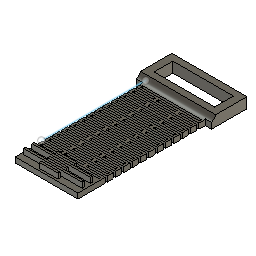
base_comp12 (Autodesk Fusion 360 design; units mm, degrees)
Autodesk Fusion 360 part; units mm, degrees
note: some values were not read from the file. Set by a fixed rule: which face or edge a step refers to.
(part 1 of 3)
sketch "Sketch1" plane through (0, 0, 0) normal (0, 0, 1) x (1, 0, 0)
  line L0 (-25, 25) -> (35, 25)
  line L1 (35, 25) -> (35, -145)
  line L2 (35, -145) -> (-25, -145)
  line L3 (-25, -145) -> (-25, 25)
  dimension "d1" = 60
  dimension "d2" = 170
  constraint perpendicular L0 L1
  constraint parallel L0 L2
  constraint parallel L1 L3
  constraint horizontal L0
  measures "d1" distance of L0.start L0.end
  measures "d2" distance of L0.start L2.end
extrude "Extrude1" add sketch "Sketch1" along normal blind 5
sketch "Sketch2" plane through (0, 0, 5) normal (0, 0, 1) x (-1, 0, 0)
  line L0 (25, 145) -> (-35, 145)
  line L1 (-35, 145) -> (-35, -25)
  line L2 (-35, -25) -> (25, -25)
  line L3 (25, -25) -> (25, 145)
  line L4 (25, -24) -> (25, -22)
  line L5 (25, -22) -> (7, -22)
  line L6 (7, -22) -> (7, -24)
  line L7 (7, -24) -> (25, -24)
  line L8 (4, -24) -> (4, -22)
  line L9 (4, -22) -> (-14, -22)
  line L10 (-14, -22) -> (-14, -24)
  line L11 (-14, -24) -> (4, -24)
  line L12 (-17, -24) -> (-17, -22)
  line L13 (-17, -22) -> (-35, -22)
  line L14 (-35, -22) -> (-35, -24)
  line L15 (-35, -24) -> (-17, -24)
  line L16 (-17, -22) -> (-35, -22)
  line L17 (-17, -24) -> (-17, -22)
  line L18 (25, -22) -> (7, -22)
  line L19 (7, -22) -> (7, -24)
  line L20 (-35, -24) -> (-17, -24)
  line L21 (4, -24) -> (4, -22)
  line L22 (-35, -22) -> (-35, -24)
  line L23 (25, -24) -> (25, -22)
  line L24 (4, -22) -> (-14, -22)
  line L25 (-14, -24) -> (4, -24)
  line L26 (-14, -22) -> (-14, -24)
  line L27 (7, -24) -> (25, -24)
  dimension "d5" = 2
  dimension "d6" = 18
  dimension "d7" = 2
  dimension "d8" = 18
  dimension "d9" = 2
  dimension "d10" = 18
  dimension "d11" = 2
  dimension "d12" = 18
  dimension "d13" = 2
  dimension "d14" = 18
  dimension "d15" = 2
  dimension "d16" = 18
  constraint perpendicular L4 L5
  constraint parallel L4 L6
  constraint parallel L5 L7
  constraint perpendicular L2 L4
  constraint coincident L3 L4.start
  constraint perpendicular L8 L9
  constraint parallel L8 L10
  constraint parallel L9 L11
  constraint perpendicular L5 L8
  constraint perpendicular L12 L13
  constraint parallel L12 L14
  constraint parallel L13 L15
  constraint parallel L1 L12
  constraint perpendicular L18 L23
  constraint parallel L19 L23
  constraint parallel L18 L27
  constraint perpendicular L21 L24
  constraint parallel L21 L26
  constraint parallel L24 L25
  constraint perpendicular L18 L21
  constraint perpendicular L16 L17
  constraint parallel L17 L22
  constraint parallel L16 L20
  measures "d5" distance of L4.start L4.end
  measures "d6" distance of L4.start L6.end
  measures "d7" distance of L8.start L8.end
  measures "d8" distance of L8.start L10.end
  measures "d9" distance of L12.start L12.end
  measures "d10" distance of L12.start L14.end
  measures "d11" distance of L4.start L4.end
  measures "d12" distance of L4.start L6.end
  measures "d13" distance of L8.end L8.start
  measures "d14" distance of L10.end L8.start
  measures "d15" distance of L12.end L12.start
  measures "d16" distance of L14.end L12.start
sketch "Sketch3" plane through (0, 0, 5) normal (0, 0, 1) x (-1, 0, 0)
  line L0 (23, -20) -> (23, -18)
  line L1 (23, -18) -> (-33, -18)
  line L2 (-33, -18) -> (-33, -20)
  line L3 (-33, -20) -> (23, -20)
  dimension "d17" = 2
  dimension "d18" = 56
  constraint perpendicular L0 L1
  constraint parallel L0 L2
  constraint parallel L1 L3
  constraint vertical L0
  measures "d17" distance of L0.start L0.end
  measures "d18" distance of L0.start L2.end
sketch "Sketch4" plane through (0, 0, 5) normal (0, 0, 1) x (-1, 0, 0)
extrude "Extrude2" cut sketch "Sketch3" against normal blind 11
extrude "Extrude3" cut sketch "Sketch2" against normal blind 26 contours L3 L4 L5 L6 L7 L18 L19 L23 L27 | L1 L12 L13 L14 L15 L16 L17 L20 L22 | L8 L9 L10 L11 L21 L24 L25 L26
sketch "Sketch5" plane through (0, 0, 5) normal (0, 0, 1) x (-1, 0, 0)
  line L0 (-17, -24) -> (-35, -24)
  line L1 (-35, -24) -> (-35, -25)
  line L2 (-35, -25) -> (25, -25)
  line L3 (25, -25) -> (25, -24)
  line L4 (25, -24) -> (7, -24)
  line L5 (7, -24) -> (7, -22)
  line L6 (7, -22) -> (25, -22)
  line L7 (25, -22) -> (25, 145)
  line L8 (25, 145) -> (-35, 145)
  line L9 (-35, 145) -> (-35, -22)
  line L10 (-35, -22) -> (-17, -22)
  line L11 (-17, -22) -> (-17, -24)
  line L12 (4, -24) -> (-14, -24)
  line L13 (-14, -24) -> (-14, -22)
  line L14 (-14, -22) -> (4, -22)
  line L15 (4, -22) -> (4, -24)
  line L16 (23, -18) -> (23, -20)
  line L17 (23, -20) -> (-33, -20)
  line L18 (-33, -20) -> (-33, -18)
  line L19 (-33, -18) -> (23, -18)
  line L20 (25, -16) -> (25, -14)
  line L21 (25, -14) -> (7, -14)
  line L22 (7, -14) -> (7, -16)
  line L23 (7, -16) -> (25, -16)
  line L24 (4, -16) -> (4, -14)
  line L25 (4, -14) -> (-14, -14)
  line L26 (-14, -14) -> (-14, -16)
  line L27 (-14, -16) -> (4, -16)
  line L28 (-17, -16) -> (-17, -14)
  line L29 (-17, -14) -> (-35, -14)
  line L30 (-35, -14) -> (-35, -16)
  line L31 (-35, -16) -> (-17, -16)
  line L32 (23, -12) -> (23, -10)
  line L33 (23, -10) -> (-33, -10)
  line L34 (-33, -10) -> (-33, -12)
  line L35 (-33, -12) -> (23, -12)
  line L36 (25, -8) -> (25, -6)
  line L37 (25, -6) -> (7, -6)
  line L38 (7, -6) -> (7, -8)
  line L39 (7, -8) -> (25, -8)
  line L40 (4, -8) -> (4, -6)
  line L41 (4, -6) -> (-14, -6)
  line L42 (-14, -6) -> (-14, -8)
  line L43 (-14, -8) -> (4, -8)
  line L44 (-17, -8) -> (-17, -6)
  line L45 (-17, -6) -> (-35, -6)
  line L46 (-35, -6) -> (-35, -8)
  line L47 (-35, -8) -> (-17, -8)
  line L48 (23, -4) -> (23, -2)
  line L49 (23, -2) -> (-33, -2)
  line L50 (-33, -2) -> (-33, -4)
  line L51 (-33, -4) -> (23, -4)
  line L52 (25, 0) -> (25, 2)
  line L53 (25, 2) -> (7, 2)
  line L54 (7, 2) -> (7, 0)
  line L55 (7, 0) -> (25, 0)
  line L56 (4, 0) -> (4, 2)
  line L57 (4, 2) -> (-14, 2)
  line L58 (-14, 2) -> (-14, 0)
  line L59 (-14, 0) -> (4, 0)
  line L60 (-17, 0) -> (-17, 2)
  line L61 (-17, 2) -> (-35, 2)
  line L62 (-35, 2) -> (-35, 0)
  line L63 (-35, 0) -> (-17, 0)
  line L64 (23, 4) -> (23, 6)
  line L65 (23, 6) -> (-33, 6)
  line L66 (-33, 6) -> (-33, 4)
  line L67 (-33, 4) -> (23, 4)
  line L68 (25, 8) -> (25, 10)
  line L69 (25, 10) -> (7, 10)
  line L70 (7, 10) -> (7, 8)
  line L71 (7, 8) -> (25, 8)
  line L72 (4, 8) -> (4, 10)
  line L73 (4, 10) -> (-14, 10)
  line L74 (-14, 10) -> (-14, 8)
  line L75 (-14, 8) -> (4, 8)
  line L76 (-17, 8) -> (-17, 10)
  line L77 (-17, 10) -> (-35, 10)
  line L78 (-35, 10) -> (-35, 8)
  line L79 (-35, 8) -> (-17, 8)
  line L80 (23, 12) -> (23, 14)
  line L81 (23, 14) -> (-33, 14)
  line L82 (-33, 14) -> (-33, 12)
  line L83 (-33, 12) -> (23, 12)
  line L84 (25, 16) -> (25, 18)
  line L85 (25, 18) -> (7, 18)
  line L86 (7, 18) -> (7, 16)
  line L87 (7, 16) -> (25, 16)
  line L88 (4, 16) -> (4, 18)
  line L89 (4, 18) -> (-14, 18)
  line L90 (-14, 18) -> (-14, 16)
  line L91 (-14, 16) -> (4, 16)
  line L92 (-17, 16) -> (-17, 18)
  line L93 (-17, 18) -> (-35, 18)
  line L94 (-35, 18) -> (-35, 16)
  line L95 (-35, 16) -> (-17, 16)
  line L96 (23, 20) -> (23, 22)
  line L97 (23, 22) -> (-33, 22)
  line L98 (-33, 22) -> (-33, 20)
  line L99 (-33, 20) -> (23, 20)
  line L100 (25, 24) -> (25, 26)
  line L101 (25, 26) -> (7, 26)
  line L102 (7, 26) -> (7, 24)
  line L103 (7, 24) -> (25, 24)
  line L104 (4, 24) -> (4, 26)
  line L105 (4, 26) -> (-14, 26)
  line L106 (-14, 26) -> (-14, 24)
  line L107 (-14, 24) -> (4, 24)
  line L108 (-17, 24) -> (-17, 26)
  line L109 (-17, 26) -> (-35, 26)
  line L110 (-35, 26) -> (-35, 24)
  line L111 (-35, 24) -> (-17, 24)
  line L112 (23, 28) -> (23, 30)
  line L113 (23, 30) -> (-33, 30)
  line L114 (-33, 30) -> (-33, 28)
  line L115 (-33, 28) -> (23, 28)
  line L116 (25, 32) -> (7, 32)
  line L117 (7, 32) -> (7, 34)
  line L118 (7, 34) -> (25, 34)
  line L119 (25, 34) -> (25, 32)
  line L120 (4, 32) -> (4, 34)
  line L121 (4, 34) -> (-14, 34)
  line L122 (-14, 34) -> (-14, 32)
  line L123 (-14, 32) -> (4, 32)
  line L124 (-17, 32) -> (-17, 34)
  line L125 (-17, 34) -> (-35, 34)
  line L126 (-35, 34) -> (-35, 32)
  line L127 (-35, 32) -> (-17, 32)
  line L128 (23, 36) -> (23, 38)
  line L129 (23, 38) -> (-33, 38)
  line L130 (-33, 38) -> (-33, 36)
  line L131 (-33, 36) -> (23, 36)
  dimension "d23" = 2
  dimension "d24" = 18
  dimension "d25" = 18
  dimension "d26" = 18
  dimension "d27" = 2
  dimension "d28" = 56
  dimension "d29" = 2
  dimension "d30" = 18
  dimension "d31" = 18
  dimension "d32" = 18
  dimension "d33" = 56
  dimension "d34" = 2
  dimension "d35" = 18
  dimension "d36" = 2
  dimension "d37" = 18
  dimension "d38" = 2
  dimension "d39" = 56
  dimension "d40" = 18
  dimension "d41" = 18
  dimension "d42" = 2
  dimension "d43" = 18
  dimension "d44" = 56
  dimension "d45" = 2
  dimension "d46" = 18
  dimension "d47" = 2
  dimension "d48" = 18
  dimension "d49" = 2
  dimension "d50" = 18
  dimension "d51" = 2
  dimension "d52" = 56
  dimension "d53" = 2
  dimension "d54" = 18
  dimension "d55" = 2
  dimension "d56" = 18
  dimension "d57" = 2
  dimension "d58" = 18
  dimension "d59" = 2
  dimension "d60" = 56
  dimension "d61" = 2
  dimension "d62" = 18
  dimension "d63" = 2
  dimension "d64" = 18
  dimension "d65" = 56
  constraint perpendicular L20 L21
  constraint parallel L20 L22
  constraint parallel L21 L23
  constraint parallel L7 L20
  constraint coincident L7 L20.start
  constraint perpendicular L24 L25
  constraint parallel L24 L26
  constraint parallel L25 L27
  constraint vertical L24
  constraint perpendicular L28 L29
  constraint parallel L28 L30
  constraint parallel L29 L31
  constraint perpendicular L27 L28
  constraint perpendicular L32 L33
  constraint parallel L32 L34
  constraint parallel L33 L35
  constraint vertical L32
  constraint perpendicular L36 L37
  constraint parallel L36 L38
  constraint parallel L37 L39
  constraint perpendicular L33 L36
  constraint coincident L7 L36.start
  constraint perpendicular L40 L41
  constraint parallel L40 L42
  constraint parallel L41 L43
  constraint perpendicular L33 L40
  constraint perpendicular L44 L45
  constraint parallel L44 L46
  constraint parallel L45 L47
  constraint perpendicular L41 L44
  constraint perpendicular L48 L49
  constraint parallel L48 L50
  constraint parallel L49 L51
  constraint perpendicular L37 L48
  constraint perpendicular L52 L53
  constraint parallel L52 L54
  constraint parallel L53 L55
  constraint perpendicular L45 L52
  constraint coincident L7 L52.start
  constraint perpendicular L56 L57
  constraint parallel L56 L58
  constraint parallel L57 L59
  constraint vertical L56
  constraint perpendicular L60 L61
  constraint parallel L60 L62
  constraint parallel L61 L63
  constraint vertical L60
  constraint perpendicular L64 L65
  constraint parallel L64 L66
  constraint parallel L65 L67
  constraint vertical L64
  constraint perpendicular L68 L69
  constraint parallel L68 L70
  constraint parallel L69 L71
  constraint coincident L7 L68.end
  constraint coincident L7 L68.start
  constraint perpendicular L72 L73
  constraint parallel L72 L74
  constraint parallel L73 L75
  constraint perpendicular L71 L72
  constraint perpendicular L76 L77
  constraint parallel L76 L78
  constraint parallel L77 L79
  constraint perpendicular L73 L76
  constraint perpendicular L80 L81
  constraint parallel L80 L82
  constraint parallel L81 L83
  constraint perpendicular L71 L80
  constraint perpendicular L84 L85
  constraint parallel L84 L86
  constraint parallel L85 L87
  constraint perpendicular L73 L84
  constraint coincident L7 L84.start
  constraint perpendicular L88 L89
  constraint parallel L88 L90
  constraint parallel L89 L91
  constraint perpendicular L85 L88
  constraint perpendicular L92 L93
  constraint parallel L92 L94
  constraint parallel L93 L95
  constraint perpendicular L81 L92
  constraint perpendicular L96 L97
  constraint parallel L96 L98
  constraint parallel L97 L99
  constraint perpendicular L85 L96
  constraint perpendicular L100 L101
  constraint parallel L100 L102
  constraint parallel L101 L103
  constraint perpendicular L97 L100
  constraint coincident L7 L100.start
  constraint perpendicular L104 L105
  constraint parallel L104 L106
  constraint parallel L105 L107
  constraint perpendicular L101 L104
  constraint perpendicular L108 L109
  constraint parallel L108 L110
  constraint parallel L109 L111
  constraint perpendicular L105 L108
  constraint perpendicular L112 L113
  constraint parallel L112 L114
  constraint parallel L113 L115
  constraint perpendicular L101 L112
  constraint horizontal L116
  constraint vertical L117
  constraint horizontal L118
  constraint vertical L119
  constraint coincident L7 L116.start
  constraint perpendicular L120 L121
  constraint parallel L120 L122
  constraint parallel L121 L123
  constraint perpendicular L113 L120
  constraint perpendicular L124 L125
  constraint parallel L124 L126
  constraint parallel L125 L127
  constraint perpendicular L121 L124
  constraint perpendicular L128 L129
  constraint parallel L128 L130
  constraint parallel L129 L131
  constraint perpendicular L118 L128
  measures "d23" distance of L20.start L20.end
  measures "d24" distance of L20.start L22.end
  measures "d25" distance of L24.start L26.end
  measures "d26" distance of L28.start L30.end
  measures "d27" distance of L32.start L32.end
  measures "d28" distance of L32.start L34.end
  measures "d29" distance of L36.start L36.end
  measures "d30" distance of L36.start L38.end
  measures "d31" distance of L40.start L42.end
  measures "d32" distance of L44.start L46.end
  measures "d33" distance of L48.start L50.end
  measures "d34" distance of L52.start L52.end
  measures "d35" distance of L52.start L54.end
  measures "d36" distance of L56.start L56.end
  measures "d37" distance of L56.start L58.end
  measures "d38" distance of L64.start L64.end
  measures "d39" distance of L64.start L66.end
  measures "d40" distance of L68.start L70.end
  measures "d41" distance of L72.start L74.end
  measures "d42" distance of L76.start L76.end
  measures "d43" distance of L76.start L78.end
  measures "d44" distance of L80.start L82.end
  measures "d45" distance of L84.start L84.end
  measures "d46" distance of L84.start L86.end
  measures "d47" distance of L88.start L88.end
  measures "d48" distance of L88.start L90.end
  measures "d49" distance of L92.start L92.end
  measures "d50" distance of L92.start L94.end
  measures "d51" distance of L96.start L96.end
  measures "d52" distance of L96.start L98.end
  measures "d53" distance of L100.start L100.end
  measures "d54" distance of L100.start L102.end
  measures "d55" distance of L104.start L104.end
  measures "d56" distance of L104.start L106.end
  measures "d57" distance of L108.start L108.end
  measures "d58" distance of L108.start L110.end
  measures "d59" distance of L112.start L112.end
  measures "d60" distance of L112.start L114.end
  measures "d61" distance of L120.start L120.end
  measures "d62" distance of L120.start L122.end
  measures "d63" distance of L124.start L124.end
  measures "d64" distance of L124.start L126.end
  measures "d65" distance of L128.start L130.end
extrude "Extrude4" cut sketch "Sketch5" against normal blind 35 contours L9 L28 L29 L30 L31 | L9 L44 L45 L46 L47 | L9 L60 L61 L62 L63 | L7 L20 L21 L22 L23 | L9 L76 L77 L78 L79 | L7 L36 L37 L38 L39 | L9 L92 L93 L94 L95 | L7 L52 L53 L54 L55 | L9 L108 L109 L110 L111 | L7 L68 L69 L70 L71 | L9 L124 L125 L126 L127 | L7 L84 L85 L86 L87 | L7 L100 L101 L102 L103 | L7 L116 L117 L118 L119 | L12 L13 L14 L15 | L16 L17 L18 L19 | L24 L25 L26 L27 | L32 L33 L34 L35 | L40 L41 L42 L43 | L48 L49 L50 L51 | L56 L57 L58 L59 | L64 L65 L66 L67 | L72 L73 L74 L75 | L80 L81 L82 L83 | L88 L89 L90 L91 | L96 L97 L98 L99 | L104 L105 L106 L107 | L112 L113 L114 L115 | L120 L121 L122 L123 | L128 L129 L130 L131
sketch "Sketch6" plane through (0, 0, 5) normal (0, 0, 1) x (-1, 0, 0)
  line L0 (25, 16) -> (7, 16)
  line L1 (7, 16) -> (7, 18)
  line L2 (7, 18) -> (25, 18)
  line L3 (25, 18) -> (25, 24)
  line L4 (25, 24) -> (7, 24)
  line L5 (7, 24) -> (7, 26)
  line L6 (7, 26) -> (25, 26)
  line L7 (25, 26) -> (25, 32)
  line L8 (25, 32) -> (7, 32)
  line L9 (7, 32) -> (7, 34)
  line L10 (7, 34) -> (25, 34)
  line L11 (25, 34) -> (25, 145)
  line L12 (25, 145) -> (-35, 145)
  line L13 (-35, 145) -> (-35, 34)
  line L14 (-35, 34) -> (-17, 34)
  line L15 (-17, 34) -> (-17, 32)
  line L16 (-17, 32) -> (-35, 32)
  line L17 (-35, 32) -> (-35, 26)
  line L18 (-35, 26) -> (-17, 26)
  line L19 (-17, 26) -> (-17, 24)
  line L20 (-17, 24) -> (-35, 24)
  line L21 (-35, 24) -> (-35, 18)
  line L22 (-35, 18) -> (-17, 18)
  line L23 (-17, 18) -> (-17, 16)
  line L24 (-17, 16) -> (-35, 16)
  line L25 (-35, 16) -> (-35, 10)
  line L26 (-35, 10) -> (-17, 10)
  line L27 (-17, 10) -> (-17, 8)
  line L28 (-17, 8) -> (-35, 8)
  line L29 (-35, 8) -> (-35, 2)
  line L30 (-35, 2) -> (-17, 2)
  line L31 (-17, 2) -> (-17, 0)
  line L32 (-17, 0) -> (-35, 0)
  line L33 (-35, 0) -> (-35, -6)
  line L34 (-35, -6) -> (-17, -6)
  line L35 (-17, -6) -> (-17, -8)
  line L36 (-17, -8) -> (-35, -8)
  line L37 (-35, -8) -> (-35, -14)
  line L38 (-35, -14) -> (-17, -14)
  line L39 (-17, -14) -> (-17, -16)
  line L40 (-17, -16) -> (-35, -16)
  line L41 (-35, -16) -> (-35, -22)
  line L42 (-35, -22) -> (-17, -22)
  line L43 (-17, -22) -> (-17, -24)
  line L44 (-17, -24) -> (-35, -24)
  line L45 (-35, -24) -> (-35, -25)
  line L46 (-35, -25) -> (25, -25)
  line L47 (25, -25) -> (25, -24)
  line L48 (25, -24) -> (7, -24)
  line L49 (7, -24) -> (7, -22)
  line L50 (7, -22) -> (25, -22)
  line L51 (25, -22) -> (25, -16)
  line L52 (25, -16) -> (7, -16)
  line L53 (7, -16) -> (7, -14)
  line L54 (7, -14) -> (25, -14)
  line L55 (25, -14) -> (25, -8)
  line L56 (25, -8) -> (7, -8)
  line L57 (7, -8) -> (7, -6)
  line L58 (7, -6) -> (25, -6)
  line L59 (25, -6) -> (25, 0)
  line L60 (25, 0) -> (7, 0)
  line L61 (7, 0) -> (7, 2)
  line L62 (7, 2) -> (25, 2)
  line L63 (25, 2) -> (25, 8)
  line L64 (25, 8) -> (7, 8)
  line L65 (7, 8) -> (7, 10)
  line L66 (7, 10) -> (25, 10)
  line L67 (25, 10) -> (25, 16)
  line L68 (23, -18) -> (23, -20)
  line L69 (23, -20) -> (-33, -20)
  line L70 (-33, -20) -> (-33, -18)
  line L71 (-33, -18) -> (23, -18)
  line L72 (4, -24) -> (-14, -24)
  line L73 (-14, -24) -> (-14, -22)
  line L74 (-14, -22) -> (4, -22)
  line L75 (4, -22) -> (4, -24)
  line L76 (23, 22) -> (23, 20)
  line L77 (23, 20) -> (-33, 20)
  line L78 (-33, 20) -> (-33, 22)
  line L79 (-33, 22) -> (23, 22)
  line L80 (23, 6) -> (23, 4)
  line L81 (23, 4) -> (-33, 4)
  line L82 (-33, 4) -> (-33, 6)
  line L83 (-33, 6) -> (23, 6)
  line L84 (23, -10) -> (23, -12)
  line L85 (23, -12) -> (-33, -12)
  line L86 (-33, -12) -> (-33, -10)
  line L87 (-33, -10) -> (23, -10)
  line L88 (4, -14) -> (4, -16)
  line L89 (4, -16) -> (-14, -16)
  line L90 (-14, -16) -> (-14, -14)
  line L91 (-14, -14) -> (4, -14)
  line L92 (4, -6) -> (4, -8)
  line L93 (4, -8) -> (-14, -8)
  line L94 (-14, -8) -> (-14, -6)
  line L95 (-14, -6) -> (4, -6)
  line L96 (4, 10) -> (4, 8)
  line L97 (4, 8) -> (-14, 8)
  line L98 (-14, 8) -> (-14, 10)
  line L99 (-14, 10) -> (4, 10)
  line L100 (4, 26) -> (4, 24)
  line L101 (4, 24) -> (-14, 24)
  line L102 (-14, 24) -> (-14, 26)
  line L103 (-14, 26) -> (4, 26)
  line L104 (4, 34) -> (4, 32)
  line L105 (4, 32) -> (-14, 32)
  line L106 (-14, 32) -> (-14, 34)
  line L107 (-14, 34) -> (4, 34)
  line L108 (4, 18) -> (4, 16)
  line L109 (4, 16) -> (-14, 16)
  line L110 (-14, 16) -> (-14, 18)
  line L111 (-14, 18) -> (4, 18)
  line L112 (4, 2) -> (4, 0)
  line L113 (4, 0) -> (-14, 0)
  line L114 (-14, 0) -> (-14, 2)
  line L115 (-14, 2) -> (4, 2)
  line L116 (23, 38) -> (23, 36)
  line L117 (23, 36) -> (-33, 36)
  line L118 (-33, 36) -> (-33, 38)
  line L119 (-33, 38) -> (23, 38)
  line L120 (23, -2) -> (23, -4)
  line L121 (23, -4) -> (-33, -4)
  line L122 (-33, -4) -> (-33, -2)
  line L123 (-33, -2) -> (23, -2)
  line L124 (23, 14) -> (23, 12)
  line L125 (23, 12) -> (-33, 12)
  line L126 (-33, 12) -> (-33, 14)
  line L127 (-33, 14) -> (23, 14)
  line L128 (23, 30) -> (23, 28)
  line L129 (23, 28) -> (-33, 28)
  line L130 (-33, 28) -> (-33, 30)
  line L131 (-33, 30) -> (23, 30)
  line L132 (25, 40) -> (25, 42)
  line L133 (25, 42) -> (7, 42)
  line L134 (7, 42) -> (7, 40)
  line L135 (7, 40) -> (25, 40)
  line L136 (4, 40) -> (4, 42)
  line L137 (4, 42) -> (-14, 42)
  line L138 (-14, 42) -> (-14, 40)
  line L139 (-14, 40) -> (4, 40)
  line L140 (-17, 40) -> (-17, 42)
  line L141 (-17, 42) -> (-35, 42)
  line L142 (-35, 42) -> (-35, 40)
  line L143 (-35, 40) -> (-17, 40)
  line L144 (23, 44) -> (23, 46.2715)
  line L145 (23, 46.2715) -> (-33, 46.2715)
  line L146 (-33, 46.2715) -> (-33, 44)
  line L147 (-33, 44) -> (23, 44)
  line L148 (25, 48) -> (7, 48)
  line L149 (7, 48) -> (7, 50)
  line L150 (7, 50) -> (25, 50)
  line L151 (25, 50) -> (25, 48)
  line L152 (4, 48) -> (4, 50)
  line L153 (4, 50) -> (-14, 50)
  line L154 (-14, 50) -> (-14, 48)
  line L155 (-14, 48) -> (4, 48)
  line L156 (-17, 48) -> (-17, 50)
  line L157 (-17, 50) -> (-35, 50)
  line L158 (-35, 50) -> (-35, 48)
  line L159 (-35, 48) -> (-17, 48)
  line L160 (23, 52) -> (23, 54)
  line L161 (23, 54) -> (-33, 54)
  line L162 (-33, 54) -> (-33, 52)
  line L163 (-33, 52) -> (23, 52)
  line L164 (25, 56) -> (25, 58)
  line L165 (25, 58) -> (7, 58)
  line L166 (7, 58) -> (7, 56)
  line L167 (7, 56) -> (25, 56)
  line L168 (4, 56) -> (4, 58)
  line L169 (4, 58) -> (-14, 58)
  line L170 (-14, 58) -> (-14, 56)
  line L171 (-14, 56) -> (4, 56)
  line L172 (-17, 56) -> (-17, 58)
  line L173 (-17, 58) -> (-35, 58)
  line L174 (-35, 58) -> (-35, 56)
  line L175 (-35, 56) -> (-17, 56)
  line L176 (23, 60) -> (23, 62)
  line L177 (23, 62) -> (-33, 62)
  line L178 (-33, 62) -> (-33, 60)
  line L179 (-33, 60) -> (23, 60)
  line L180 (25, 64) -> (25, 66)
  line L181 (25, 66) -> (7, 66)
  line L182 (7, 66) -> (7, 64)
  line L183 (7, 64) -> (25, 64)
  line L184 (4, 64) -> (4, 66)
  line L185 (4, 66) -> (-14, 66)
  line L186 (-14, 66) -> (-14, 64)
  line L187 (-14, 64) -> (4, 64)
  line L188 (-17, 64) -> (-17, 66)
  line L189 (-17, 66) -> (-35, 66)
  line L190 (-35, 66) -> (-35, 64)
  line L191 (-35, 64) -> (-17, 64)
  line L192 (23, 68) -> (23, 70)
  line L193 (23, 70) -> (-33, 70)
  line L194 (-33, 70) -> (-33, 68)
  line L195 (-33, 68) -> (23, 68)
  line L196 (25, 72) -> (25, 74)
  line L197 (25, 74) -> (7, 74)
  line L198 (7, 74) -> (7, 72)
  line L199 (7, 72) -> (25, 72)
  line L200 (4, 72) -> (4, 74)
  line L201 (4, 74) -> (-14, 74)
  line L202 (-14, 74) -> (-14, 72)
  line L203 (-14, 72) -> (4, 72)
  line L204 (-17, 72) -> (-17, 74)
  line L205 (-17, 74) -> (-35, 74)
  line L206 (-35, 74) -> (-35, 72)
  line L207 (-35, 72) -> (-17, 72)
  line L208 (23, 76) -> (23, 78)
  line L209 (23, 78) -> (-33, 78)
  line L210 (-33, 78) -> (-33, 76)
  line L211 (-33, 76) -> (23, 76)
  line L212 (25, 80) -> (25, 82)
  line L213 (25, 82) -> (7, 82)
  line L214 (7, 82) -> (7, 80)
  line L215 (7, 80) -> (25, 80)
  line L216 (4, 80) -> (4, 82)
  line L217 (4, 82) -> (-14, 82)
  line L218 (-14, 82) -> (-14, 80)
  line L219 (-14, 80) -> (4, 80)
  line L220 (-17, 80) -> (-17, 82)
  line L221 (-17, 82) -> (-35, 82)
  line L222 (-35, 82) -> (-35, 80)
  line L223 (-35, 80) -> (-17, 80)
  line L224 (23, 84) -> (23, 86)
  line L225 (23, 86) -> (-33, 86)
  line L226 (-33, 86) -> (-33, 84)
  line L227 (-33, 84) -> (23, 84)
  line L228 (7, 88) -> (7, 90)
  line L229 (7, 90) -> (25, 90)
  line L230 (25, 90) -> (25, 88)
  line L231 (25, 88) -> (7, 88)
  line L232 (4, 88) -> (4, 90)
  line L233 (4, 90) -> (-14, 90)
  line L234 (-14, 90) -> (-14, 88)
  line L235 (-14, 88) -> (4, 88)
  line L236 (-17, 88) -> (-17, 90)
  line L237 (-17, 90) -> (-35, 90)
  line L238 (-35, 90) -> (-35, 88)
  line L239 (-35, 88) -> (-17, 88)
  line L240 (-33, 92) -> (-33, 94)
  line L241 (-33, 94) -> (23, 94)
  line L242 (23, 94) -> (23, 92)
  line L243 (23, 92) -> (-33, 92)
  line L244 (25, 96) -> (7, 96)
  line L245 (7, 96) -> (7, 98)
  line L246 (7, 98) -> (25, 98)
  line L247 (25, 98) -> (25, 96)
  line L248 (4, 96) -> (4, 98)
  line L249 (4, 98) -> (-14, 98)
  line L250 (-14, 98) -> (-14, 96)
  line L251 (-14, 96) -> (4, 96)
  line L252 (-17, 96) -> (-17, 98)
  line L253 (-17, 98) -> (-35, 98)
  line L254 (-35, 98) -> (-35, 96)
  line L255 (-35, 96) -> (-17, 96)
  line L256 (23, 100) -> (23, 102)
  line L257 (23, 102) -> (-32.9874, 102)
  line L258 (-32.9874, 102) -> (-32.9874, 100)
  line L259 (-32.9874, 100) -> (23, 100)
  line L260 (25, 104) -> (25, 106)
  line L261 (25, 106) -> (7, 106)
  line L262 (7, 106) -> (7, 104)
  line L263 (7, 104) -> (25, 104)
  line L264 (4, 104) -> (4, 106)
  line L265 (4, 106) -> (-14, 106)
  line L266 (-14, 106) -> (-14, 104)
  line L267 (-14, 104) -> (4, 104)
  line L268 (-17, 104) -> (-17, 106)
  line L269 (-17, 106) -> (-35, 106)
  line L270 (-35, 106) -> (-35, 104)
  line L271 (-35, 104) -> (-17, 104)
  line L272 (23, 108) -> (23, 110)
  line L273 (23, 110) -> (-33, 110)
  line L274 (-33, 110) -> (-33, 108)
  line L275 (-33, 108) -> (23, 108)
  line L276 (25, 112) -> (25, 114)
  line L277 (25, 114) -> (7, 114)
  line L278 (7, 114) -> (7, 112)
  line L279 (7, 112) -> (25, 112)
  line L280 (4, 112) -> (4, 114)
  line L281 (4, 114) -> (-14, 114)
  line L282 (-14, 114) -> (-14, 112)
  line L283 (-14, 112) -> (4, 112)
  line L284 (-17, 112) -> (-17, 114)
  line L285 (-17, 114) -> (-35, 114)
  line L286 (-35, 114) -> (-35, 112)
  line L287 (-35, 112) -> (-17, 112)
  line L288 (23, 116) -> (-33, 116)
  line L289 (-33, 116) -> (-33, 118)
  line L290 (-33, 118) -> (23, 118)
  line L291 (23, 118) -> (23, 116)
  dimension "d68" = 2
  dimension "d69" = 18
  dimension "d70" = 18
  dimension "d71" = 18
  dimension "d72" = 56
  dimension "d73" = 2
  dimension "d74" = 18
  dimension "d75" = 2
  dimension "d76" = 18
  dimension "d77" = 2
  dimension "d78" = 56
  dimension "d79" = 2
  dimension "d80" = 18
  dimension "d81" = 18
  dimension "d82" = 56
  dimension "d83" = 56
  dimension "d84" = 2
  dimension "d85" = 56
  dimension "d86" = 18
  dimension "d87" = 56
  dimension "d88" = 56
  dimension "d89" = 2
  dimension "d90" = 2
  dimension "d91" = 18
  dimension "d92" = 56
  dimension "d93" = 18
  dimension "d94" = 18
  constraint perpendicular L132 L133
  constraint parallel L132 L134
  constraint parallel L133 L135
  constraint parallel L11 L132
  constraint coincident L11 L132.start
  constraint perpendicular L136 L137
  constraint parallel L136 L138
  constraint parallel L137 L139
  constraint perpendicular L119 L136
  constraint perpendicular L140 L141
  constraint parallel L140 L142
  constraint parallel L141 L143
  constraint perpendicular L119 L140
  constraint perpendicular L144 L145
  constraint parallel L144 L146
  constraint parallel L145 L147
  constraint perpendicular L133 L144
  constraint horizontal L148
  constraint vertical L149
  constraint horizontal L150
  constraint vertical L151
  constraint coincident L11 L148.start
  constraint perpendicular L152 L153
  constraint parallel L152 L154
  constraint parallel L153 L155
  constraint perpendicular L145 L152
  constraint perpendicular L156 L157
  constraint parallel L156 L158
  constraint parallel L157 L159
  constraint perpendicular L145 L156
  constraint perpendicular L160 L161
  constraint parallel L160 L162
  constraint parallel L161 L163
  constraint perpendicular L145 L160
  constraint perpendicular L164 L165
  constraint parallel L164 L166
  constraint parallel L165 L167
  constraint perpendicular L148 L164
  constraint coincident L11 L164.start
  constraint perpendicular L168 L169
  constraint parallel L168 L170
  constraint parallel L169 L171
  constraint perpendicular L167 L168
  constraint perpendicular L172 L173
  constraint parallel L172 L174
  constraint parallel L173 L175
  constraint perpendicular L161 L172
  constraint perpendicular L176 L177
  constraint parallel L176 L178
  constraint parallel L177 L179
  constraint perpendicular L147 L176
  constraint perpendicular L180 L181
  constraint parallel L180 L182
  constraint parallel L181 L183
  constraint coincident L11 L180.end
  constraint coincident L11 L180.start
  constraint perpendicular L184 L185
  constraint parallel L184 L186
  constraint parallel L185 L187
  constraint perpendicular L181 L184
  constraint perpendicular L188 L189
  constraint parallel L188 L190
  constraint parallel L189 L191
  constraint perpendicular L185 L188
  constraint perpendicular L192 L193
  constraint parallel L192 L194
  constraint parallel L193 L195
  constraint perpendicular L189 L192
  constraint perpendicular L196 L197
  constraint parallel L196 L198
  constraint parallel L197 L199
  constraint coincident L11 L196.end
  constraint coincident L11 L196.start
  constraint perpendicular L200 L201
  constraint parallel L200 L202
  constraint parallel L201 L203
  constraint perpendicular L197 L200
  constraint perpendicular L204 L205
  constraint parallel L204 L206
  constraint parallel L205 L207
  constraint perpendicular L201 L204
  constraint perpendicular L208 L209
  constraint parallel L208 L210
  constraint parallel L209 L211
  constraint perpendicular L197 L208
  constraint perpendicular L212 L213
  constraint parallel L212 L214
  constraint parallel L213 L215
  constraint coincident L11 L212.end
  constraint coincident L11 L212.start
  constraint perpendicular L216 L217
  constraint parallel L216 L218
  constraint parallel L217 L219
  constraint perpendicular L209 L216
  constraint perpendicular L220 L221
  constraint parallel L220 L222
  constraint parallel L221 L223
  constraint perpendicular L217 L220
  constraint perpendicular L224 L225
  constraint parallel L224 L226
  constraint parallel L225 L227
  constraint perpendicular L221 L224
  constraint perpendicular L228 L229
  constraint parallel L228 L230
  constraint parallel L229 L231
  constraint perpendicular L225 L228
  constraint perpendicular L232 L233
  constraint parallel L232 L234
  constraint parallel L233 L235
  constraint perpendicular L229 L232
  constraint perpendicular L236 L237
  constraint parallel L236 L238
  constraint parallel L237 L239
  constraint perpendicular L233 L236
  constraint perpendicular L240 L241
  constraint parallel L240 L242
  constraint parallel L241 L243
  constraint perpendicular L237 L240
  constraint horizontal L244
  constraint vertical L245
  constraint horizontal L246
  constraint vertical L247
  constraint coincident L11 L244.start
  constraint perpendicular L248 L249
  constraint parallel L248 L250
  constraint parallel L249 L251
  constraint perpendicular L241 L248
  constraint perpendicular L252 L253
  constraint parallel L252 L254
  constraint parallel L253 L255
  constraint perpendicular L249 L252
  constraint perpendicular L256 L257
  constraint parallel L256 L258
  constraint parallel L257 L259
  constraint perpendicular L255 L256
  constraint perpendicular L260 L261
  constraint parallel L260 L262
  constraint parallel L261 L263
  constraint perpendicular L259 L260
  constraint coincident L11 L260.start
  constraint perpendicular L264 L265
  constraint parallel L264 L266
  constraint parallel L265 L267
  constraint perpendicular L261 L264
  constraint perpendicular L268 L269
  constraint parallel L268 L270
  constraint parallel L269 L271
  constraint perpendicular L265 L268
  constraint perpendicular L272 L273
  constraint parallel L272 L274
  constraint parallel L273 L275
  constraint perpendicular L265 L272
  constraint perpendicular L276 L277
  constraint parallel L276 L278
  constraint parallel L277 L279
  constraint coincident L11 L276.end
  constraint coincident L11 L276.start
  constraint perpendicular L280 L281
  constraint parallel L280 L282
  constraint parallel L281 L283
  constraint perpendicular L265 L280
  constraint perpendicular L284 L285
  constraint parallel L284 L286
  constraint parallel L285 L287
  constraint perpendicular L265 L284
  constraint horizontal L288
  constraint vertical L289
  constraint horizontal L290
  constraint vertical L291
  measures "d68" distance of L132.start L132.end
  measures "d69" distance of L132.start L134.end
  measures "d70" distance of L136.start L138.end
  measures "d71" distance of L140.start L142.end
  measures "d72" distance of L144.start L146.end
  measures "d73" distance of L152.start L152.end
  measures "d74" distance of L152.start L154.end
  measures "d75" distance of L156.start L156.end
  measures "d76" distance of L156.start L158.end
  measures "d77" distance of L160.start L160.end
  measures "d78" distance of L160.start L162.end
  measures "d79" distance of L164.start L164.end
  measures "d80" distance of L164.start L166.end
  measures "d81" distance of L168.start L170.end
  measures "d82" distance of L176.start L178.end
  measures "d83" distance of L192.start L194.end
  measures "d84" distance of L208.start L208.end
  measures "d85" distance of L208.start L210.end
  measures "d86" distance of L212.start L214.end
  measures "d87" distance of L224.start L226.end
  measures "d88" distance of L240.start L242.end
  measures "d89" distance of L260.start L260.end
  measures "d90" distance of L268.start L268.end
  measures "d91" distance of L268.start L270.end
  measures "d92" distance of L272.start L274.end
  measures "d93" distance of L280.start L282.end
  measures "d94" distance of L284.start L286.end
extrude "Extrude5" cut sketch "Sketch6" against normal blind 50 contours L11 L132 L133 L134 L135 | L11 L148 L149 L150 L151 | L11 L164 L165 L166 L167 | L11 L180 L181 L182 L183 | L11 L196 L197 L198 L199 | L11 L212 L213 L214 L215 | L11 L228 L229 L230 L231 | L11 L244 L245 L246 L247 | L11 L260 L261 L262 L263 | L11 L276 L277 L278 L279 | L13 L284 L285 L286 L287 | L13 L268 L269 L270 L271 | L13 L252 L253 L254 L255 | L13 L236 L237 L238 L239 | L13 L220 L221 L222 L223 | L13 L204 L205 L206 L207 | L13 L188 L189 L190 L191 | L13 L172 L173 L174 L175 | L13 L156 L157 L158 L159 | L13 L140 L141 L142 L143 | L136 L137 L138 L139 | L144 L145 L146 L147 | L152 L153 L154 L155 | L160 L161 L162 L163 | L168 L169 L170 L171 | L176 L177 L178 L179 | L184 L185 L186 L187 | L192 L193 L194 L195 | L200 L201 L202 L203 | L208 L209 L210 L211 | L216 L217 L218 L219 | L224 L225 L226 L227 | L232 L233 L234 L235 | L240 L241 L242 L243 | L248 L249 L250 L251 | L256 L257 L258 L259 | L264 L265 L266 L267 | L272 L273 L274 L275 | L280 L281 L282 L283 | L288 L289 L290 L291
sketch "Sketch7" plane through (0, 0, 5) normal (0, 0, 1) x (-1, 0, 0)
  line L0 (-17, 56) -> (-35, 56)
  line L1 (-35, 56) -> (-35, 50)
  line L2 (-35, 50) -> (-17, 50)
  line L3 (-17, 50) -> (-17, 48)
  line L4 (-17, 48) -> (-35, 48)
  line L5 (-35, 48) -> (-35, 42)
  line L6 (-35, 42) -> (-17, 42)
  line L7 (-17, 42) -> (-17, 40)
  line L8 (-17, 40) -> (-35, 40)
  line L9 (-35, 40) -> (-35, 34)
  line L10 (-35, 34) -> (-17, 34)
  line L11 (-17, 34) -> (-17, 32)
  line L12 (-17, 32) -> (-35, 32)
  line L13 (-35, 32) -> (-35, 26)
  line L14 (-35, 26) -> (-17, 26)
  line L15 (-17, 26) -> (-17, 24)
  line L16 (-17, 24) -> (-35, 24)
  line L17 (-35, 24) -> (-35, 18)
  line L18 (-35, 18) -> (-17, 18)
  line L19 (-17, 18) -> (-17, 16)
  line L20 (-17, 16) -> (-35, 16)
  line L21 (-35, 16) -> (-35, 10)
  line L22 (-35, 10) -> (-17, 10)
  line L23 (-17, 10) -> (-17, 8)
  line L24 (-17, 8) -> (-35, 8)
  line L25 (-35, 8) -> (-35, 2)
  line L26 (-35, 2) -> (-17, 2)
  line L27 (-17, 2) -> (-17, 0)
  line L28 (-17, 0) -> (-35, 0)
  line L29 (-35, 0) -> (-35, -6)
  line L30 (-35, -6) -> (-17, -6)
  line L31 (-17, -6) -> (-17, -8)
  line L32 (-17, -8) -> (-35, -8)
  line L33 (-35, -8) -> (-35, -14)
  line L34 (-35, -14) -> (-17, -14)
  line L35 (-17, -14) -> (-17, -16)
  line L36 (-17, -16) -> (-35, -16)
  line L37 (-35, -16) -> (-35, -22)
  line L38 (-35, -22) -> (-17, -22)
  line L39 (-17, -22) -> (-17, -24)
  line L40 (-17, -24) -> (-35, -24)
  line L41 (-35, -24) -> (-35, -25)
  line L42 (-35, -25) -> (25, -25)
  line L43 (25, -25) -> (25, -24)
  line L44 (25, -24) -> (7, -24)
  line L45 (7, -24) -> (7, -22)
  line L46 (7, -22) -> (25, -22)
  line L47 (25, -22) -> (25, -16)
  line L48 (25, -16) -> (7, -16)
  line L49 (7, -16) -> (7, -14)
  line L50 (7, -14) -> (25, -14)
  line L51 (25, -14) -> (25, -8)
  line L52 (25, -8) -> (7, -8)
  line L53 (7, -8) -> (7, -6)
  line L54 (7, -6) -> (25, -6)
  line L55 (25, -6) -> (25, 0)
  line L56 (25, 0) -> (7, 0)
  line L57 (7, 0) -> (7, 2)
  line L58 (7, 2) -> (25, 2)
  line L59 (25, 2) -> (25, 8)
  line L60 (25, 8) -> (7, 8)
  line L61 (7, 8) -> (7, 10)
  line L62 (7, 10) -> (25, 10)
  line L63 (25, 10) -> (25, 16)
  line L64 (25, 16) -> (7, 16)
  line L65 (7, 16) -> (7, 18)
  line L66 (7, 18) -> (25, 18)
  line L67 (25, 18) -> (25, 24)
  line L68 (25, 24) -> (7, 24)
  line L69 (7, 24) -> (7, 26)
  line L70 (7, 26) -> (25, 26)
  line L71 (25, 26) -> (25, 32)
  line L72 (25, 32) -> (7, 32)
  line L73 (7, 32) -> (7, 34)
  line L74 (7, 34) -> (25, 34)
  line L75 (25, 34) -> (25, 40)
  line L76 (25, 40) -> (7, 40)
  line L77 (7, 40) -> (7, 42)
  line L78 (7, 42) -> (25, 42)
  line L79 (25, 42) -> (25, 48)
  line L80 (25, 48) -> (7, 48)
  line L81 (7, 48) -> (7, 50)
  line L82 (7, 50) -> (25, 50)
  line L83 (25, 50) -> (25, 56)
  line L84 (25, 56) -> (7, 56)
  line L85 (7, 56) -> (7, 58)
  line L86 (7, 58) -> (25, 58)
  line L87 (25, 58) -> (25, 64)
  line L88 (25, 64) -> (7, 64)
  line L89 (7, 64) -> (7, 66)
  line L90 (7, 66) -> (25, 66)
  line L91 (25, 66) -> (25, 72)
  line L92 (25, 72) -> (7, 72)
  line L93 (7, 72) -> (7, 74)
  line L94 (7, 74) -> (25, 74)
  line L95 (25, 74) -> (25, 80)
  line L96 (25, 80) -> (7, 80)
  line L97 (7, 80) -> (7, 82)
  line L98 (7, 82) -> (25, 82)
  line L99 (25, 82) -> (25, 88)
  line L100 (25, 88) -> (7, 88)
  line L101 (7, 88) -> (7, 90)
  line L102 (7, 90) -> (25, 90)
  line L103 (25, 90) -> (25, 96)
  line L104 (25, 96) -> (7, 96)
  line L105 (7, 96) -> (7, 98)
  line L106 (7, 98) -> (25, 98)
  line L107 (25, 98) -> (25, 104)
  line L108 (25, 104) -> (7, 104)
  line L109 (7, 104) -> (7, 106)
  line L110 (7, 106) -> (25, 106)
  line L111 (25, 106) -> (25, 112)
  line L112 (25, 112) -> (7, 112)
  line L113 (7, 112) -> (7, 114)
  line L114 (7, 114) -> (25, 114)
  line L115 (25, 114) -> (25, 145)
  line L116 (25, 145) -> (-35, 145)
  line L117 (-35, 145) -> (-35, 114)
  line L118 (-35, 114) -> (-17, 114)
  line L119 (-17, 114) -> (-17, 112)
  line L120 (-17, 112) -> (-35, 112)
  line L121 (-35, 112) -> (-35, 106)
  line L122 (-35, 106) -> (-17, 106)
  line L123 (-17, 106) -> (-17, 104)
  line L124 (-17, 104) -> (-35, 104)
  line L125 (-35, 104) -> (-35, 98)
  line L126 (-35, 98) -> (-17, 98)
  line L127 (-17, 98) -> (-17, 96)
  line L128 (-17, 96) -> (-35, 96)
  line L129 (-35, 96) -> (-35, 90)
  line L130 (-35, 90) -> (-17, 90)
  line L131 (-17, 90) -> (-17, 88)
  line L132 (-17, 88) -> (-35, 88)
  line L133 (-35, 88) -> (-35, 82)
  line L134 (-35, 82) -> (-17, 82)
  line L135 (-17, 82) -> (-17, 80)
  line L136 (-17, 80) -> (-35, 80)
  line L137 (-35, 80) -> (-35, 74)
  line L138 (-35, 74) -> (-17, 74)
  line L139 (-17, 74) -> (-17, 72)
  line L140 (-17, 72) -> (-35, 72)
  line L141 (-35, 72) -> (-35, 66)
  line L142 (-35, 66) -> (-17, 66)
  line L143 (-17, 66) -> (-17, 64)
  line L144 (-17, 64) -> (-35, 64)
  line L145 (-35, 64) -> (-35, 58)
  line L146 (-35, 58) -> (-17, 58)
  line L147 (-17, 58) -> (-17, 56)
  line L148 (23, 30) -> (23, 28)
  line L149 (23, 28) -> (-33, 28)
  line L150 (-33, 28) -> (-33, 30)
  line L151 (-33, 30) -> (23, 30)
  line L152 (23, 14) -> (23, 12)
  line L153 (23, 12) -> (-33, 12)
  line L154 (-33, 12) -> (-33, 14)
  line L155 (-33, 14) -> (23, 14)
  line L156 (23, -2) -> (23, -4)
  line L157 (23, -4) -> (-33, -4)
  line L158 (-33, -4) -> (-33, -2)
  line L159 (-33, -2) -> (23, -2)
  line L160 (23, 38) -> (23, 36)
  line L161 (23, 36) -> (-33, 36)
  line L162 (-33, 36) -> (-33, 38)
  line L163 (-33, 38) -> (23, 38)
  line L164 (4, 2) -> (4, 0)
  line L165 (4, 0) -> (-14, 0)
  line L166 (-14, 0) -> (-14, 2)
  line L167 (-14, 2) -> (4, 2)
  line L168 (4, 18) -> (4, 16)
  line L169 (4, 16) -> (-14, 16)
  line L170 (-14, 16) -> (-14, 18)
  line L171 (-14, 18) -> (4, 18)
  line L172 (4, 34) -> (4, 32)
  line L173 (4, 32) -> (-14, 32)
  line L174 (-14, 32) -> (-14, 34)
  line L175 (-14, 34) -> (4, 34)
  line L176 (4, 26) -> (4, 24)
  line L177 (4, 24) -> (-14, 24)
  line L178 (-14, 24) -> (-14, 26)
  line L179 (-14, 26) -> (4, 26)
  line L180 (4, 10) -> (4, 8)
  line L181 (4, 8) -> (-14, 8)
  line L182 (-14, 8) -> (-14, 10)
  line L183 (-14, 10) -> (4, 10)
  line L184 (4, -6) -> (4, -8)
  line L185 (4, -8) -> (-14, -8)
  line L186 (-14, -8) -> (-14, -6)
  line L187 (-14, -6) -> (4, -6)
  line L188 (4, -14) -> (4, -16)
  line L189 (4, -16) -> (-14, -16)
  line L190 (-14, -16) -> (-14, -14)
  line L191 (-14, -14) -> (4, -14)
  line L192 (23, -10) -> (23, -12)
  line L193 (23, -12) -> (-33, -12)
  line L194 (-33, -12) -> (-33, -10)
  line L195 (-33, -10) -> (23, -10)
  line L196 (23, 6) -> (23, 4)
  line L197 (23, 4) -> (-33, 4)
  line L198 (-33, 4) -> (-33, 6)
  line L199 (-33, 6) -> (23, 6)
  line L200 (23, 22) -> (23, 20)
  line L201 (23, 20) -> (-33, 20)
  line L202 (-33, 20) -> (-33, 22)
  line L203 (-33, 22) -> (23, 22)
  line L204 (4, -24) -> (-14, -24)
  line L205 (-14, -24) -> (-14, -22)
  line L206 (-14, -22) -> (4, -22)
  line L207 (4, -22) -> (4, -24)
  line L208 (23, -18) -> (23, -20)
  line L209 (23, -20) -> (-33, -20)
  line L210 (-33, -20) -> (-33, -18)
  line L211 (-33, -18) -> (23, -18)
  line L212 (4, 58) -> (4, 56)
  line L213 (4, 56) -> (-14, 56)
  line L214 (-14, 56) -> (-14, 58)
  line L215 (-14, 58) -> (4, 58)
  line L216 (23, 86) -> (23, 84)
  line L217 (23, 84) -> (-33, 84)
  line L218 (-33, 84) -> (-33, 86)
  line L219 (-33, 86) -> (23, 86)
  line L220 (23, 46.2715) -> (23, 44)
  line L221 (23, 44) -> (-33, 44)
  line L222 (-33, 44) -> (-33, 46.2715)
  line L223 (-33, 46.2715) -> (23, 46.2715)
  line L224 (4, 98) -> (4, 96)
  line L225 (4, 96) -> (-14, 96)
  line L226 (-14, 96) -> (-14, 98)
  line L227 (-14, 98) -> (4, 98)
  line L228 (4, 114) -> (4, 112)
  line L229 (4, 112) -> (-14, 112)
  line L230 (-14, 112) -> (-14, 114)
  line L231 (-14, 114) -> (4, 114)
  line L232 (23, 110) -> (23, 108)
  line L233 (23, 108) -> (-33, 108)
  line L234 (-33, 108) -> (-33, 110)
  line L235 (-33, 110) -> (23, 110)
  line L236 (23, 70) -> (23, 68)
  line L237 (23, 68) -> (-33, 68)
  line L238 (-33, 68) -> (-33, 70)
  line L239 (-33, 70) -> (23, 70)
  line L240 (4, 42) -> (4, 40)
  line L241 (4, 40) -> (-14, 40)
  line L242 (-14, 40) -> (-14, 42)
  line L243 (-14, 42) -> (4, 42)
  line L244 (4, 82) -> (4, 80)
  line L245 (4, 80) -> (-14, 80)
  line L246 (-14, 80) -> (-14, 82)
  line L247 (-14, 82) -> (4, 82)
  line L248 (-33, 116) -> (-33, 118)
  line L249 (-33, 118) -> (23, 118)
  line L250 (23, 118) -> (23, 116)
  line L251 (23, 116) -> (-33, 116)
  line L252 (23, 62) -> (23, 60)
  line L253 (23, 60) -> (-33, 60)
  line L254 (-33, 60) -> (-33, 62)
  line L255 (-33, 62) -> (23, 62)
  line L256 (4, 74) -> (4, 72)
  line L257 (4, 72) -> (-14, 72)
  line L258 (-14, 72) -> (-14, 74)
  line L259 (-14, 74) -> (4, 74)
  line L260 (4, 90) -> (4, 88)
  line L261 (4, 88) -> (-14, 88)
  line L262 (-14, 88) -> (-14, 90)
  line L263 (-14, 90) -> (4, 90)
  line L264 (4, 50) -> (4, 48)
  line L265 (4, 48) -> (-14, 48)
  line L266 (-14, 48) -> (-14, 50)
  line L267 (-14, 50) -> (4, 50)
  line L268 (23, 102) -> (23, 100)
  line L269 (23, 100) -> (-32.9874, 100)
  line L270 (-32.9874, 100) -> (-32.9874, 102)
  line L271 (-32.9874, 102) -> (23, 102)
  line L272 (4, 106) -> (4, 104)
  line L273 (4, 104) -> (-14, 104)
  line L274 (-14, 104) -> (-14, 106)
  line L275 (-14, 106) -> (4, 106)
  line L276 (4, 66) -> (4, 64)
  line L277 (4, 64) -> (-14, 64)
  line L278 (-14, 64) -> (-14, 66)
  line L279 (-14, 66) -> (4, 66)
  line L280 (23, 54) -> (23, 52)
  line L281 (23, 52) -> (-33, 52)
  line L282 (-33, 52) -> (-33, 54)
  line L283 (-33, 54) -> (23, 54)
  line L284 (-33, 94) -> (23, 94)
  line L285 (23, 94) -> (23, 92)
  line L286 (23, 92) -> (-33, 92)
  line L287 (-33, 92) -> (-33, 94)
  line L288 (23, 78) -> (23, 76)
  line L289 (23, 76) -> (-33, 76)
  line L290 (-33, 76) -> (-33, 78)
  line L291 (-33, 78) -> (23, 78)
  line L292 (25, 120) -> (25, 122)
  line L293 (25, 122) -> (7, 122)
  line L294 (7, 122) -> (7, 120)
  line L295 (7, 120) -> (25, 120)
  line L296 (4, 120) -> (4, 122)
  line L297 (4, 122) -> (-14, 122)
  line L298 (-14, 122) -> (-14, 120)
  line L299 (-14, 120) -> (4, 120)
  line L300 (-17, 120) -> (-17, 122)
  line L301 (-17, 122) -> (-35, 122)
  line L302 (-35, 122) -> (-35, 120)
  line L303 (-35, 120) -> (-17, 120)
  line L304 (23, 124) -> (23, 126)
  line L305 (23, 126) -> (-33, 126)
  line L306 (-33, 126) -> (-33, 124)
  line L307 (-33, 124) -> (23, 124)
  line L308 (25, 128) -> (25, 130)
  line L309 (25, 130) -> (7, 130)
  line L310 (7, 130) -> (7, 128)
  line L311 (7, 128) -> (25, 128)
  line L312 (4, 128) -> (4, 130)
  line L313 (4, 130) -> (-14, 130)
  line L314 (-14, 130) -> (-14, 128)
  line L315 (-14, 128) -> (4, 128)
  line L316 (-17, 128) -> (-17, 130)
  line L317 (-17, 130) -> (-35, 130)
  line L318 (-35, 130) -> (-35, 128)
  line L319 (-35, 128) -> (-17, 128)
  line L320 (23, 132) -> (23, 134)
  line L321 (23, 134) -> (-33, 134)
  line L322 (-33, 134) -> (-33, 132)
  line L323 (-33, 132) -> (23, 132)
  line L324 (25, 136) -> (25, 138)
  line L325 (25, 138) -> (7, 138)
  line L326 (7, 138) -> (7, 136)
  line L327 (7, 136) -> (25, 136)
  line L328 (4, 136) -> (4, 138)
  line L329 (4, 138) -> (-14, 138)
  line L330 (-14, 138) -> (-14, 136)
  line L331 (-14, 136) -> (4, 136)
  line L332 (-17, 136) -> (-17, 138)
  line L333 (-17, 138) -> (-35, 138)
  line L334 (-35, 138) -> (-35, 136)
  line L335 (-35, 136) -> (-17, 136)
  line L336 (23, 140) -> (23, 142)
  line L337 (23, 142) -> (-33, 142)
  line L338 (-33, 142) -> (-33, 140)
  line L339 (-33, 140) -> (23, 140)
  dimension "d97" = 18
  constraint perpendicular L292 L293
  constraint parallel L292 L294
  constraint parallel L293 L295
  constraint coincident L115 L292.end
  constraint coincident L115 L292.start
  constraint perpendicular L296 L297
  constraint parallel L296 L298
  constraint parallel L297 L299
  constraint perpendicular L293 L296
  constraint perpendicular L300 L301
  constraint parallel L300 L302
  constraint parallel L301 L303
  constraint perpendicular L297 L300
  constraint perpendicular L304 L305
  constraint parallel L304 L306
  constraint parallel L305 L307
  constraint perpendicular L301 L304
  constraint perpendicular L308 L309
  constraint parallel L308 L310
  constraint parallel L309 L311
  constraint coincident L115 L308.end
  constraint coincident L115 L308.start
  constraint perpendicular L312 L313
  constraint parallel L312 L314
  constraint parallel L313 L315
  constraint perpendicular L309 L312
  constraint perpendicular L316 L317
  constraint parallel L316 L318
  constraint parallel L317 L319
  constraint perpendicular L313 L316
  constraint perpendicular L320 L321
  constraint parallel L320 L322
  constraint parallel L321 L323
  constraint perpendicular L313 L320
  constraint perpendicular L324 L325
  constraint parallel L324 L326
  constraint parallel L325 L327
  constraint coincident L115 L324.end
  constraint coincident L115 L324.start
  constraint perpendicular L328 L329
  constraint parallel L328 L330
  constraint parallel L329 L331
  constraint perpendicular L325 L328
  constraint perpendicular L332 L333
  constraint parallel L332 L334
  constraint parallel L333 L335
  constraint perpendicular L329 L332
  constraint perpendicular L336 L337
  constraint parallel L336 L338
  constraint parallel L337 L339
  constraint perpendicular L333 L336
  measures "d97" distance of L292.start L294.end
extrude "Extrude6" cut sketch "Sketch7" against normal blind 43 contours L117 L300 L301 L302 L303 | L117 L316 L317 L318 L319 | L117 L332 L333 L334 L335 | L115 L324 L325 L326 L327 | L115 L308 L309 L310 L311 | L115 L292 L293 L294 L295 | L296 L297 L298 L299 | L304 L305 L306 L307 | L312 L313 L314 L315 | L320 L321 L322 L323 | L328 L329 L330 L331 | L336 L337 L338 L339
extrude "Extrude7" add 1 faces at (15, -145, 1.6667) along direction (0, -1, 0) blind 5